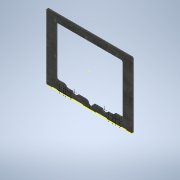
# Autodesk Inventor part: PRO FRAME
Saved by Autodesk Inventor 2023 (Build 270158000, 158)
## iProperties
Created: 2019-05-27
Part Number: PRO FRAME
Material: Steel
Document SubType Name: Modeling
Designer: Parker
Density: 7.85 g/cm^3
Appearance: Plate
Author: Parker
Autodesk Inventor part; units mm, degrees
ref_plane "YZ Plane" through (0, 0, 0) normal (1, 0, 0) x (0, 1, 0)
ref_plane "XZ Plane" through (0, 0, 0) normal (0, 1, 0) x (-1, 0, 0)
ref_plane "XY Plane" through (0, 0, 0) normal (0, 0, 1) x (1, 0, 0)
sketch "Sketch13" plane through (0, 0, 0) normal (0, 0, 1) x (1, 0, 0)
  line L0 (-245, -187.5) -> (245, -187.5)
  line L1 (245, -187.5) -> (245, 187.5)
  line L2 (245, 187.5) -> (-245, 187.5)
  line L3 (-245, 187.5) -> (-245, -187.5)
  line L4 (-245, -187.5) -> (245, 187.5) construction
  line L5 (245, -187.5) -> (-245, 187.5) construction
  point P0 (0, 0)
  dimension "d93" = 490
  dimension "d94" = 375
  constraints: 12 end point, 2 midpoint, 2 parallel, 1 horizontal, 1 perpendicular
  measures "d93" distance of L1.end L2.end
  measures "d94" distance of L2.end L0.start
extrude "Extrusion6" add sketch "Sketch13" along normal blind 6.35
sketch "Critical Positions" plane through (0, 0, 6.35) normal (0, 0, 1) x (1, 0, 0)
  line L0 (-245, -187.5) -> (245, -187.5) projected
  line L1 (0, -187.5) -> (0, -161.7604) construction
  point P0 (0, 0)
  point P1 (-85, -145.5)
  point P2 (85, -145.5)
  point P3 (-110.4, -182.64)
  point P4 (110.4, -182.64)
  point P5 (-110.4, -159.44)
  point P6 (-133.6, -182.64)
  point P7 (-133.6, -159.44)
  point P8 (110.4, -182.64)
  point P9 (110.4, -159.44)
  point P10 (133.6, -182.64)
  point P11 (133.6, -159.44)
  point P12 (-170.6, -159.44)
  point P13 (-170.6, -182.64)
  point P14 (-147.4, -159.44)
  point P15 (-147.4, -182.64)
  point P16 (147.4, -182.64)
  point P17 (147.4, -159.44)
  point P18 (170.6, -182.64)
  point P19 (170.6, -159.44)
  point P20 (147.4, -182.64)
  dimension "d97" = 170
  dimension "d98" = 85
  dimension "d99" = 42
  dimension "d104" = 220.8
  dimension "d105" = 110.4
  dimension "d106" = 4.86
  dimension "d109" = 23.2
  dimension "d112" = 23.2
  dimension "d124" = 37
  dimension "d131" = 37
  constraints: 4 symmetric about line, 3 horizontal, 2 end point, 2 horizontal alignment, 2 vertical, 1 midpoint, 12 other
  measures "d97" distance of point (85, -145.5) point (-85, -145.5)
  measures "d98" horizontal distance of point (0, 0) point (85, -145.5)
  measures "d99" distance from line of point (85, -145.5) L0
  measures "d104" distance of point (-110.4, -182.64) point (110.4, -182.64)
  measures "d105" horizontal distance of point (0, 0) point (-110.4, -182.64)
  measures "d106" distance from line of L0 point (-110.4, -182.64)
  measures "d109" distance of point (-110.4, -182.64) point (-110.4, -159.44)
  measures "d112" distance of point (-110.4, -182.64) point (-133.6, -182.64)
  measures "d124" distance of point (-133.6, -159.44) point (-170.6, -159.44)
  measures "d131" distance of point (110.4, -182.64) point (147.4, -182.64)
sketch "Rail Clearance" plane through (0, 0, 6.35) normal (0, 0, 1) x (1, 0, 0)
  circle A0 centre (-85, -145.5) radius 17.5
  circle A1 centre (85, -145.5) radius 17.5
  point P0 (0, 0)
  dimension "d100" = 35
  dimension "d101" = 35
  constraints: 2 centre point, 2 coincident
  measures "d100" diameter of A0
  measures "d101" diameter of A1
extrude "Extrusion7" cut sketch "Rail Clearance" against normal blind 6.35
sketch "Sketch16" plane through (0, 0, 6.35) normal (0, 0, 1) x (1, 0, 0)
  point P0 (0, 0)
  point P1 (-133.6, -159.44)
  point P2 (-110.4, -159.44)
  point P3 (-110.4, -182.64)
  point P4 (-133.6, -182.64)
  point P5 (110.4, -159.44)
  point P6 (110.4, -182.64)
  point P7 (133.6, -182.64)
  point P8 (133.6, -159.44)
  point P9 (-147.4, -182.64)
  point P10 (-170.6, -182.64)
  point P11 (-170.6, -159.44)
  point P12 (-147.4, -159.44)
  point P13 (147.4, -159.44)
  point P14 (170.6, -159.44)
  point P15 (170.6, -182.64)
  point P16 (147.4, -182.64)
hole "Aluminum Extrusion Mounting Holes" at (-133.6, -159.44, 6.35) at (-110.4, -159.44, 6.35) at (-110.4, -182.64, 6.35) at (-133.6, -182.64, 6.35) at (110.4, -159.44, 6.35) at (110.4, -182.64, 6.35) at (133.6, -182.64, 6.35) at (133.6, -159.44, 6.35) at (-147.4, -182.64, 6.35) at (-170.6, -182.64, 6.35) at (-170.6, -159.44, 6.35) at (147.4, -159.44, 6.35) at (170.6, -182.64, 6.35) at (170.6, -159.44, 6.35) at (147.4, -182.64, 6.35) at (-147.4, -159.44, 6.35) direction (0, 0, -1) diameter 5.4 end through all clearance for "Socket Head Cap Screw" size "M5" standard "Ansi Metric M Profile"
sketch "Sketch17" plane through (0, 0, 6.35) normal (0, 0, 1) x (1, 0, 0)
  line L0 (-13.6434, -151.5) -> (-6, -172.5)
  line L1 (-6, -172.5) -> (6, -172.5)
  line L2 (6, -172.5) -> (13.6434, -151.5)
  line L3 (-245, -187.5) -> (245, -187.5) projected
  line L4 (-68.5607, -151.5) -> (68.5607, -151.5)
  circle A0 centre (-85, -145.5) radius 17.5 projected
  circle A1 centre (85, -145.5) radius 17.5 projected
  line L5 (6, -172.5) -> (13, -172.5)
  line L6 (13, -172.5) -> (20.6434, -151.5)
  point P0 (0, 0)
  dimension "d136" = 12
  dimension "d137" = 15
  dimension "d138" = 6
  dimension "d139" = 110
  dimension "d140" = 110
  dimension "d141" = 36
  dimension "d299" = 7
  constraints: 12 end point, 3 horizontal, 3 point on line, 1 parallel, 4 other
  measures "d136" distance of L0.end L1.end
  measures "d137" distance between parallel lines of L3 L1
  measures "d138" horizontal distance of point (0, 0) L1.end
  measures "d139" angle of L1 L0
  measures "d140" angle of L2 L1
  measures "d141" distance between parallel lines of L3 L4
  measures "d299" distance of L1.end L5.end
extrude "Extrusion8" cut sketch "Sketch17" against normal blind 6.35 contours L4 L2 L1 L0 | L4 L6 L5 L2
sketch "Sketch18" plane through (0, 0, 6.35) normal (0, 0, 1) x (1, 0, 0)
  line L0 (-190, 146.5) -> (-190, -137.5)
  line L1 (190, 146.5) -> (190, -137.5)
  line L2 (-245, 187.5) -> (-245, -187.5) projected
  line L3 (245, -187.5) -> (245, 187.5) projected
  line L4 (-190, 146.5) -> (190, 146.5)
  line L5 (-13.6434, -151.5) -> (20.6434, -151.5) projected
  line L6 (-145, -137.5) -> (-190, -137.5)
  line L7 (145, -137.5) -> (190, -137.5)
  line L8 (-245, -187.5) -> (245, -187.5) projected
  line L9 (-13.6434, -151.5) -> (-131, -151.5)
  line L10 (13.6434, -151.5) -> (131, -151.5)
  line L11 (131, -151.5) -> (145, -137.5)
  line L12 (-131, -151.5) -> (-145, -137.5)
  point P0 (0, 0)
  dimension "d144" = 55
  dimension "d145" = 55
  dimension "d146" = 298
  dimension "d147" = 100
  dimension "d148" = 100
  dimension "d149" = 50
  dimension "d150" = 50
  dimension "d151" = 45
  dimension "d152" = 45
  constraints: 18 end point, 5 horizontal, 2 vertical
  measures "d144" distance between parallel lines of L2 L0
  measures "d145" distance between parallel lines of L3 L1
  measures "d146" distance between parallel lines of L5 L4
  measures "d147" distance from line of L2 L6.start
  measures "d148" distance from line of L3 L7.start
  measures "d149" distance between parallel lines of L8 L6
  measures "d150" distance between parallel lines of L8 L7
  measures "d151" angle of L9 L12
  measures "d152" angle of L10 L11
extrude "Extrusion9" cut sketch "Sketch18" against normal through all
fillet "Fillet3" radius 7 8 edges at (-68.5607, -151.5, 3.175) (-101.4393, -151.5, 3.175) (68.5607, -151.5, 3.175) (101.4393, -151.5, 3.175) (131, -151.5, 3.175) (145, -137.5, 3.175) (-145, -137.5, 3.175) (-131, -151.5, 3.175)
fillet "Fillet4" radius 10 4 edges at (-190, -137.5, 3.175) (-190, 146.5, 3.175) (190, 146.5, 3.175) (190, -137.5, 3.175)
fillet "Fillet5" radius 15 2 edges at (-13.6434, -151.5, 3.175) (20.6434, -151.5, 3.175)
fillet "Fillet6" radius 3 2 edges at (13, -172.5, 3.175) (-6, -172.5, 3.175)
sketch "Sketch19" plane through (0, 0, 6.35) normal (0, 0, 1) x (1, 0, 0)
  line L0 (245, 187.5) -> (-245, 187.5) projected
  point P0 (0, 0)
  point P1 (-235, 177.5)
  point P2 (-215, 177.5)
  point P3 (-235, -142.5)
  point P4 (-215, -142.5)
  point P5 (-225, -162.5)
  point P6 (215, -142.5)
  point P7 (235, -142.5)
  point P8 (225, -162.5)
  point P9 (235, 177.5)
  point P10 (215, 177.5)
  dimension "d159" = 20
  dimension "d160" = 20
  dimension "d161" = 470
  dimension "d162" = 20
  dimension "d163" = 20
  dimension "d164" = 20
  dimension "d165" = 10
  dimension "d166" = 20
  dimension "d167" = 10
  dimension "d168" = 320
  dimension "d169" = 320
  dimension "d172" = 215
  dimension "d173" = 10
  constraints: 5 horizontal alignment, 2 vertical alignment
  measures "d159" distance of point (235, 177.5) point (215, 177.5)
  measures "d160" distance of point (-235, 177.5) point (-215, 177.5)
  measures "d161" distance of point (235, 177.5) point (-235, 177.5)
  measures "d162" distance of point (-215, -142.5) point (-235, -142.5)
  measures "d163" distance of point (235, -142.5) point (215, -142.5)
  measures "d164" vertical distance of point (-235, -142.5) point (-225, -162.5)
  measures "d165" horizontal distance of point (-235, -142.5) point (-225, -162.5)
  measures "d166" vertical distance of point (225, -162.5) point (215, -142.5)
  measures "d167" horizontal distance of point (215, -142.5) point (225, -162.5)
  measures "d168" distance of point (235, 177.5) point (235, -142.5)
  measures "d169" distance of point (-235, -142.5) point (-235, 177.5)
  measures "d172" horizontal distance of point (215, 177.5) point (0, 0)
  measures "d173" distance from line of L0 point (-235, 177.5)
hole "Hole6" at (-235, 177.5, 6.35) at (-215, 177.5, 6.35) at (-235, -142.5, 6.35) at (-215, -142.5, 6.35) at (-225, -162.5, 6.35) at (215, -142.5, 6.35) at (235, -142.5, 6.35) at (225, -162.5, 6.35) at (235, 177.5, 6.35) at (215, 177.5, 6.35) direction (0, 0, -1) diameter 2.2 end through all
chamfer "Chamfer1" distance 5 angle 45 2 edges at (-245, 187.5, 3.175) (245, 187.5, 3.175)
sketch "Sketch20" plane through (0, 0, 6.35) normal (0, 0, 1) x (1, 0, 0)
  line L0 (245, -187.5) -> (245, 182.5) projected
  point P0 (0, 0)
  point P1 (215, 100.3448)
  point P2 (215, -49.6552)
  dimension "d184" = 150
  dimension "d185" = 30
  constraints: 1 vertical alignment
  measures "d184" distance of point (215, -49.655) point (215, 100.345)
  measures "d185" distance from line of L0 point (215, 100.345)
hole "Hole7" at (215, 100.3448, 6.35) at (215, -49.6552, 6.35) direction (0, 0, -1) diameter 4.3 end through all clearance for "Socket Head Cap Screw" size "M4" standard "Ansi Metric M Profile"
sketch "Sketch21" plane through (0, 0, 6.35) normal (0, 0, 1) x (1, 0, 0)
  line L0 (0, 0) -> (-33.4173, 0) construction
  line L1 (0, 0) -> (0, -1.6733) construction
  line L2 (-41, 0) -> (-41, -1.6733) construction
  line L3 (0, -16.5) -> (0, -18.1733) construction
  line L4 (-41, -16.5) -> (-41, -18.1733) construction
  line L5 (240, 187.5) -> (-240, 187.5) projected
  point P0 (-167.5, 171)
  point P1 (-208.5, 171)
  point P2 (-167.5, 154.5)
  point P3 (-208.5, 154.5)
  point P4 (167.5, 171)
  point P5 (208.5, 171)
  point P6 (167.5, 154.5)
  point P7 (208.5, 154.5)
  dimension "d197" = 41
  dimension "d200" = 16.5
  dimension "d203" = 16.5
  dimension "d204" = 167.5
  constraints: 10 end point, 4 symmetric about line, 2 horizontal, 2 vertical, 1 collinear, 11 other
  measures "d197" distance of L0.start L2.start
  measures "d200" distance of L0.start L3.start
  measures "d203" distance from line of L5 point (-208.5, 171)
  measures "d204" horizontal distance of L0.start point (-167.5, 171)
hole "Hole8" at (-167.5, 171, 6.35) at (-208.5, 171, 6.35) at (-167.5, 154.5, 6.35) at (-208.5, 154.5, 6.35) at (208.5, 154.5, 6.35) at (167.5, 154.5, 6.35) at (208.5, 171, 6.35) at (167.5, 171, 6.35) direction (0, 0, -1) diameter 2.2 end through all
chamfer "Chamfer2" distance 5 angle 45 2 edges at (-245, -187.5, 3.175) (245, -187.5, 3.175)
sketch "Sketch22" plane through (0, 0, 6.35) normal (0, 0, 1) x (1, 0, 0)
  line L0 (-240, -187.5) -> (240, -187.5) projected
  line L1 (-215, -187.5) -> (-210, -182.5)
  line L2 (-210, -182.5) -> (-182, -182.5)
  line L3 (-182, -182.5) -> (-177, -187.5)
  line L4 (0, 0) -> (0, -238.2091) construction
  line L5 (215, -187.5) -> (210, -182.5)
  line L6 (210, -182.5) -> (182, -182.5)
  line L7 (182, -182.5) -> (177, -187.5)
  dimension "d215" = 5
  dimension "d216" = 45
  dimension "d217" = 45
  dimension "d218" = 25
  dimension "d219" = 28
  constraints: 14 end point, 4 symmetric about line, 2 point on line, 1 parallel, 1 vertical
  measures "d215" distance between parallel lines of L0 L2
  measures "d216" angle of L0 L1
  measures "d217" angle of L0 L3
  measures "d218" distance of L0.start L1.start
  measures "d219" distance of L1.end L2.end
extrude "Extrusion10" cut sketch "Sketch22" against normal blind 6.35
sketch "Sketch23" plane through (0, 0, 6.35) normal (0, 0, 1) x (1, 0, 0)
  line L0 (-177, -187.5) -> (177, -187.5) projected
  line L1 (-104, -187.5) -> (-99, -182.5)
  line L2 (-99, -182.5) -> (-38.8994, -182.5)
  line L3 (-38.8994, -182.5) -> (-33.8994, -187.5)
  line L4 (33.8994, -187.5) -> (38.8994, -182.5)
  line L5 (38.8994, -182.5) -> (99, -182.5)
  line L6 (99, -182.5) -> (104, -187.5)
  circle A0 centre (-110.4, -182.64) radius 2.7 projected
  circle A1 centre (110.4, -182.64) radius 2.7 projected
  arc A2 (3.8994, -172.5) -> (6.7185, -170.5261) centre (3.8994, -169.5) ccw
  arc A3 (-6.7185, -170.5261) -> (-3.8994, -172.5) centre (-3.8994, -169.5) ccw
  arc A4 (10.8994, -172.5) -> (13.7185, -170.5261) centre (10.8994, -169.5) ccw projected
  point P0 (0, 0)
  dimension "d222" = 45
  dimension "d223" = 45
  dimension "d224" = 45
  dimension "d225" = 5
  dimension "d226" = 5
  dimension "d227" = 6.4
  dimension "d228" = 6.4
  dimension "d229" = 30
  dimension "d230" = 30
  dimension "d300" = 7
  constraints: 12 end point, 4 point on circle, 4 point on line, 2 centre point, 1 horizontal, 1 parallel, 1 perpendicular
  measures "d222" angle of L0 L1
  measures "d223" angle of L0 L3
  measures "d224" angle of L0 L4
  measures "d225" distance between parallel lines of L0 L2
  measures "d226" distance between parallel lines of L0 L5
  measures "d227" horizontal distance of A0.centre L1.start
  measures "d228" horizontal distance of A1.centre L6.end
  measures "d229" horizontal distance of A2.centre L4.start
  measures "d230" horizontal distance of A3.centre L3.end
  measures "d300" distance of A2.centre A4.centre
extrude "Extrusion11" cut sketch "Sketch23" against normal blind 6.35 contours L1 L2 L3 L0 | L4 L5 L6 L0
sketch "Sketch24" plane through (0, 0, 6.35) normal (0, 0, 1) x (1, 0, 0)
  line L0 (240, 187.5) -> (-240, 187.5) projected
  point P0 (0, 0)
  point P1 (-130, 167.5)
  point P2 (-30, 167.5)
  point P3 (70, 167.5)
  dimension "d233" = 20
  dimension "d234" = 130
  dimension "d237" = 100
  constraints: 1 horizontal, 2 other
  measures "d233" distance from line of L0 point (-130, 167.5)
  measures "d234" horizontal distance of point (0, 0) point (-130, 167.5)
  measures "d237" distance of point (-130, 167.5) point (-30, 167.5)
hole "Hole9" at (-130, 167.5, 6.35) at (-30, 167.5, 6.35) at (70, 167.5, 6.35) direction (0, 0, -1) diameter 2.2 end through all
sketch "Sketch25" plane through (0, 0, 6.35) normal (0, 0, 1) x (1, 0, 0)
  line L0 (182, -182.5) -> (210, -182.5) projected
  line L1 (104, -187.5) -> (177, -187.5) projected
  circle A0 centre (170.6, -182.64) radius 2.7 projected
  line L2 (-33.8994, -187.5) -> (33.8994, -187.5) projected
  line L3 (-33.8994, -187.5) -> (33.8994, -187.5) projected
  line L4 (0, -187.5) -> (0, -122.5808)
  point P0 (0, 0)
  point P1 (209, -178.5)
  point P2 (200, -178.5)
  point P3 (180.6, -179)
  point P4 (180.6, -170)
  point P5 (100.4, -179)
  point P6 (100.4, -170)
  point P7 (32.8994, -182.5)
  point P8 (32.8994, -173.5)
  point P9 (-209, -178.5)
  point P10 (-200, -178.5)
  point P11 (-180.6, -179)
  point P12 (-180.6, -170)
  point P13 (-100.4, -179)
  point P14 (-100.4, -170)
  point P15 (-32.8994, -182.5)
  point P16 (-32.8994, -173.5)
  dimension "d249" = 9
  dimension "d250" = 4
  dimension "d251" = 1
  dimension "d259" = 9
  dimension "d260" = 8.5
  dimension "d261" = 10
  dimension "d264" = 80.2
  dimension "d269" = 9
  dimension "d270" = 5
  dimension "d271" = 1
  constraints: 8 symmetric about line, 2 end point, 2 vertical alignment, 1 horizontal, 1 horizontal alignment, 1 midpoint, 1 vertical, 2 other
  measures "d249" distance of point (209, -178.5) point (200, -178.5)
  measures "d250" distance from line of L0 point (209, -178.5)
  measures "d251" horizontal distance of point (209, -178.5) L0.end
  measures "d259" distance of point (180.6, -170) point (180.6, -179)
  measures "d260" distance from line of point (180.6, -179) L1
  measures "d261" horizontal distance of A0.centre point (180.6, -179)
  measures "d264" distance of point (180.6, -179) point (100.4, -179)
  measures "d269" distance of point (32.899, -182.5) point (32.899, -173.5)
  measures "d270" distance from line of L2 point (32.899, -182.5)
  measures "d271" horizontal distance of point (32.899, -182.5) L2.end
hole "Hole10" at (209, -178.5, 6.35) at (200, -178.5, 6.35) at (180.6, -170, 6.35) at (100.4, -179, 6.35) at (100.4, -170, 6.35) at (180.6, -179, 6.35) at (32.8994, -182.5, 6.35) at (32.8994, -173.5, 6.35) at (-32.8994, -182.5, 6.35) at (-32.8994, -173.5, 6.35) at (-100.4, -179, 6.35) at (-100.4, -170, 6.35) at (-180.6, -179, 6.35) at (-180.6, -170, 6.35) at (-200, -178.5, 6.35) at (-209, -178.5, 6.35) direction (0, 0, -1) diameter 3.2 end through all
sketch "Sketch27" plane through (0, 0, 6.35) normal (0, 0, 1) x (1, 0, 0)
  point P0 (0, 0)
  point P1 (-228, 110.5)
  point P2 (-196.5, 89)
  point P3 (-228, 68)
  point P4 (-239.5, 89)
  point P5 (-239.3, 1.2)
  point P6 (-238, -18)
  point P7 (-200, -18)
  point P8 (-196, -5.2)
  point P9 (-239.3, -80)
  point P10 (-196, -80)
  point P11 (-237.7, -112)
  point P12 (-200, -112)
  dimension "d272" = 200
  dimension "d273" = 37.7
  dimension "d274" = 43.3
  dimension "d275" = 196
  dimension "d276" = 80
  dimension "d277" = 112
  dimension "d278" = 38
  dimension "d279" = 18
  dimension "d280" = 200
  dimension "d281" = 43.3
  dimension "d282" = 6.4
  dimension "d283" = 196
  dimension "d284" = 5.2
  dimension "d285" = 68
  dimension "d286" = 43
  dimension "d287" = 11.5
  dimension "d288" = 21.5
  dimension "d289" = 11.5
  dimension "d290" = 21
  dimension "d291" = 228
  constraints: 4 horizontal alignment
  measures "d272" horizontal distance of point (0, 0) point (-200, -112)
  measures "d273" distance of point (-200, -112) point (-237.7, -112)
  measures "d274" distance of point (-196, -80) point (-239.3, -80)
  measures "d275" horizontal distance of point (0, 0) point (-196, -80)
  measures "d276" vertical distance of point (0, 0) point (-196, -80)
  measures "d277" vertical distance of point (0, 0) point (-200, -112)
  measures "d278" distance of point (-238, -18) point (-200, -18)
  measures "d279" vertical distance of point (0, 0) point (-200, -18)
  measures "d280" horizontal distance of point (0, 0) point (-200, -18)
  measures "d281" horizontal distance of point (-196, -5.2) point (-239.3, 1.2)
  measures "d282" vertical distance of point (-239.3, 1.2) point (-196, -5.2)
  measures "d283" horizontal distance of point (0, 0) point (-196, -5.2)
  measures "d284" vertical distance of point (-196, -5.2) point (0, 0)
  measures "d285" vertical distance of point (0, 0) point (-228, 68)
  measures "d286" distance of point (-196.5, 89) point (-239.5, 89)
  measures "d287" horizontal distance of point (-239.5, 89) point (-228, 110.5)
  measures "d288" vertical distance of point (-228, 110.5) point (-239.5, 89)
  measures "d289" horizontal distance of point (-239.5, 89) point (-228, 68)
  measures "d290" vertical distance of point (-196.5, 89) point (-228, 68)
  measures "d291" horizontal distance of point (0, 0) point (-228, 68)
hole "Hole11" at (-228, 110.5, 6.35) at (-196.5, 89, 6.35) at (-228, 68, 6.35) at (-239.5, 89, 6.35) at (-239.3, 1.2, 6.35) at (-238, -18, 6.35) at (-200, -18, 6.35) at (-196, -5.2, 6.35) at (-239.3, -80, 6.35) at (-196, -80, 6.35) at (-237.7, -112, 6.35) at (-200, -112, 6.35) direction (0, 0, -1) diameter 2.2 end through all
sketch "Sketch28" plane through (0, 0, 6.35) normal (0, 0, 1) x (1, 0, 0)
  circle A0 centre (235, 145.9255) radius 2.75
  circle A1 centre (220.0015, 145.7106) radius 2.75
  circle A2 centre (222.4999, 180.75) radius 2.75
  line L0 (240, 187.5) -> (-240, 187.5) projected
  line L1 (245, -182.5) -> (245, 182.5) projected
  point P0 (0, 0)
  dimension "d308" = 35.0394
  dimension "d309" = 14.9985
  dimension "d310" = 0.2149
  dimension "d311" = 2.4984
  dimension "d312" = 6.75
  dimension "d313" = 10
  constraints: 3 centre point
  measures "d308" vertical distance of A1.centre A2.centre
  measures "d309" horizontal distance of A0.centre A1.centre
  measures "d310" vertical distance of A1.centre A0.centre
  measures "d311" horizontal distance of A2.centre A1.centre
  measures "d312" distance from line of L0 A2.centre
  measures "d313" distance from line of L1 A0.centre
hole "Hole12" at (220.0015, 145.7106, 6.35) at (235, 145.9255, 6.35) at (222.4999, 180.75, 6.35) direction (0, 0, -1) diameter 2.2 end through all
sketch "Sketch29" plane through (0, 0, 6.35) normal (0, 0, 1) x (1, 0, 0)
  circle A0 centre (-30, 167.5) radius 1.1 projected
  line L0 (0, 167.5) -> (0, 191.2993)
  point P0 (0, 0)
  point P1 (30, 167.5)
  constraints: 2 end point, 1 horizontal alignment, 1 symmetric about line, 1 vertical
hole "Hole13" at (0, 167.5, 6.35) at (30, 167.5, 6.35) direction (0, 0, -1) diameter 2.2 end through all
body "Solid3"
